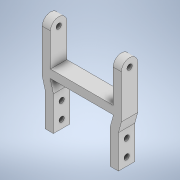
# Autodesk Inventor part: Стойка для камеры
Saved by Autodesk Inventor 2020 (Build 240168000, 168)
## iProperties
Created: 2021-04-12
Part Number: Стойка для камеры
Material: Типовые
Document SubType Name: Обычные детали
Designer: Антон
Density: 1 g/cm^3
Appearance: По умолчанию
Sheet Metal Rule: По умолчанию
Author: Антон
Autodesk Inventor part; units mm, degrees
ref_plane "YZ Plane" through (0, 0, 0) normal (1, 0, 0) x (0, 1, 0)
ref_plane "XZ Plane" through (0, 0, 0) normal (0, 1, 0) x (-1, 0, 0)
ref_plane "XY Plane" through (0, 0, 0) normal (0, 0, 1) x (1, 0, 0)
sketch "Эскиз1" plane through (0, 0, 0) normal (0, 0, 1) x (1, 0, 0)
  line L0 (0, 0) -> (5, 0)
  line L1 (5, 0) -> (5, 18)
  line L2 (5, 18) -> (0, 18)
  line L3 (0, 18) -> (0, 0)
  line L4 (0, 0) -> (24.15, 0)
  line L5 (24.15, 0) -> (24.15, -5)
  line L6 (24.15, -5) -> (0, -5)
  line L7 (0, -5) -> (0, 0)
  dimension "d0" = 5
  dimension "d1" = 18
  dimension "d2" = 24.15
  dimension "d3" = 5
  constraints: 16 end point, 4 parallel, 2 horizontal, 2 perpendicular
  measures "d0" distance of L2.end L1.end
  measures "d1" distance of L1.end L0.end
  measures "d2" distance of L5.end L6.end
  measures "d3" distance of L4.end L5.end
extrude "Выдавливание1" add sketch "Эскиз1" along normal blind 10
sketch "Эскиз4" plane through (0, 18, 0) normal (0, 1, 0) x (1, 0, 0)
  line L0 (0, 0) -> (0, -10) projected
  line L1 (0, 0) -> (0, -10) projected
  line L2 (5, 0) -> (0, 0) projected
  line L3 (0, 0) -> (0, -10) projected
  line L4 (5, -10) -> (0, -10) projected
  line L5 (5, 0) -> (5, -10) projected
extrude "Выдавливание2" add sketch "Эскиз4" along normal blind 7.2
fillet "Сопряжение1" radius 5 2 edges at (2.5, 25.2, 10) (2.5, 25.2, 0)
sketch "Эскиз5" plane through (5, 0, 10) normal (1, 0, 0) x (0, 0, -1)
  line L0 (0, -5) -> (0, -5) projected
  line L1 (10, -5) -> (10, -5) projected
  arc A0 (10, 20.2) -> (0, 20.2) centre (5, 20.2) ccw projected
  point P0 (10, 0)
  constraints: 2 other
hole "Отверстие2" at (5, 20.2, 5) direction (-1, 0, 0) diameter 3.2 depth 5
mirror "Зеркальное отражение1" about plane through (24.15, -5, 0) normal (1, 0, 0)
sketch "Эскиз9" plane through (0, 0, 0) normal (0, 0, -1) x (-1, 0, 0)
  line L0 (-48.3, 20.2) -> (-48.3, -5) projected
  line L1 (-48.3, -5) -> (-43.3, -5)
  line L2 (-43.3, -5) -> (-43.3, -6.325)
  line L3 (-43.3, -6.325) -> (-48.3, -6.325)
  line L4 (-48.3, -6.325) -> (-48.3, -5)
  line L5 (-48.3, -6.325) -> (-43.4788, -5)
  line L6 (-43.4788, -5) -> (-41.5, -12.2)
  line L7 (-41.5, -12.2) -> (-46.3212, -13.525)
  line L8 (-46.3212, -13.525) -> (-48.3, -6.325)
  line L9 (-41.5, -12.2) -> (-46.5, -12.2)
  line L10 (-46.5, -12.2) -> (-46.5, -33.2)
  line L11 (-46.5, -33.2) -> (-41.5, -33.2)
  line L12 (-41.5, -33.2) -> (-41.5, -12.2)
  line L13 (0, -5) -> (-48.3, -5) projected
  point P0 (0, 0)
  point P1 (-43.3, -5.6504)
  point P2 (-46.5, -12.8746)
  dimension "d39" = 5
  dimension "d45" = 5
  dimension "d47" = 5
  dimension "d66" = 28.2
  dimension "d68" = 21
  dimension "d70" = 1.8
  constraints: 24 end point, 6 parallel, 3 perpendicular, 1 horizontal, 1 point on line
  measures "d39" distance of L2.end L3.end
  measures "d45" distance between parallel lines of L6 L8
  measures "d47" distance between parallel lines of L12 L10
  measures "d66" distance between parallel lines of L1 L11
  measures "d68" distance of L9.end L10.end
  measures "d70" distance between parallel lines of L4 L10
extrude "Выдавливание4" add sketch "Эскиз9" against normal blind 10
sketch "Эскиз10" plane through (46.5, -33.2, 0) normal (1, 0, 0) x (0, 0, -1)
  line L0 (0, 0) -> (-10, 0) projected
  line L1 (-5, 0) -> (-5, 5)
  line L2 (-5, 5) -> (-5, 15)
  point P0 (0, 33.2)
  dimension "d48" = 5
  dimension "d49" = 10
  constraints: 4 end point, 2 vertical, 1 midpoint
  measures "d48" distance of L1.start L1.end
  measures "d49" distance of L1.end L2.end
hole "Отверстие5" at (46.5, -18.2, 5) at (46.5, -28.2, 5) direction (-1, 0, 0) diameter 3.2 end through all
ref_plane "РабПлоскость1" through (24.15, 20.2, 5) normal (1, 0, 0) x (0, 0, -1)
mirror "Зеркальное отражение2" about plane through (24.15, 20.2, 5) normal (1, 0, 0) of "Выдавливание4", "Отверстие5"
equation "\"d63\" = Толщина"
equation "\"Радиус_гибки\" = Толщина"
equation "\"Ширина_просечки\" = Толщина"
equation "\"Глубина_просечки\" = 0.5 * Толщина"
equation "\"Размер_просечки\" = 4 * Толщина"
equation "\"Мин_остаток\" = 2 * Толщина"
equation "\"Радиус_перехода\" = Радиус_гибки"
equation "\"Радиус_Якоби\" = Толщина"
equation "\"Размер_зазора\" = Толщина"
equation "\"Толщина\" = 0.5"
